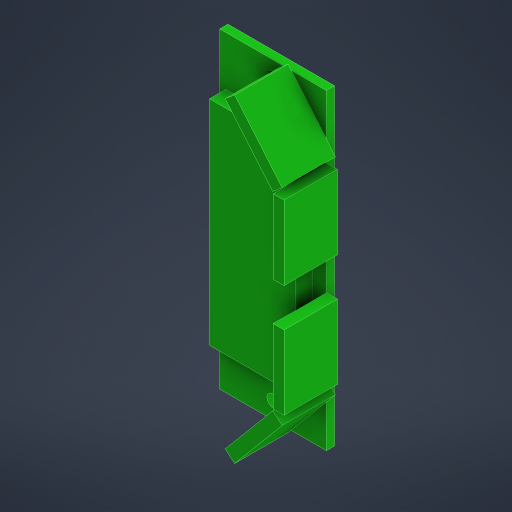
# Autodesk Inventor part: płytka_pcb
Saved by Autodesk Inventor 2023.4 (Build 274418000, 418)
## iProperties
Created: 2025-10-31
Part Number: płytka_pcb
Material: Tworzywo sztuczne ABS
Document SubType Name: Modeling
Designer: Jakub Borsukiewicz
Density: 1.06 g/cm^3
Appearance: Ciemnozielona
Author: Jakub Borsukiewicz
Autodesk Inventor part; units mm, degrees
ref_plane "YZ Plane" through (0, 0, 0) normal (1, 0, 0) x (0, 1, 0)
ref_plane "XZ Plane" through (0, 0, 0) normal (0, 1, 0) x (-1, 0, 0)
ref_plane "XY Plane" through (0, 0, 0) normal (0, 0, 1) x (1, 0, 0)
sketch "Szkic1" plane through (0, 0, 0) normal (0, 0, 1) x (1, 0, 0)
  line L0 (0, -7.6) -> (0, 45.6) projected
  line L1 (-5.2, 0) -> (31.2, 0) projected
  line L2 (0, 0) -> (26, 0)
  line L3 (26, 0) -> (26, 38)
  line L4 (26, 38) -> (0, 38)
  line L5 (0, 38) -> (0, 0)
  circle A0 centre (13, 34) radius 1.5
  point P0 (0, 38)
  dimension "d0" = 26
  dimension "d1" = 38
  dimension "d2" = 3
  dimension "d3" = 4
  dimension "d4" = 13
  constraints: 8 end point, 2 parallel, 1 centre point, 1 horizontal, 1 perpendicular
  measures "d0" distance of L3.end L4.end
  measures "d1" distance of L2.end L3.end
  measures "d2" diameter of A0
  measures "d3" distance from line of L4 A0.centre
  measures "d4" distance from line of L5 A0.centre
extrude "Wyciągnięcie proste1" add sketch "Szkic1" along normal blind 2
sketch "Szkic2" plane through (0, 0, 2) normal (0, 0, 1) x (1, 0, 0)
  line L0 (0, 38) -> (0, 0) projected
  line L1 (0, 0) -> (26, 0) projected
  line L2 (26, 0) -> (26, 38) projected
  line L3 (26, 38) -> (0, 38) projected
  circle A0 centre (13, 34) radius 1.5 projected
  line L4 (0, 0) -> (26, 0) projected
  line L5 (1.5, 0) -> (22.5, 0)
  line L6 (22.5, 0) -> (22.5, 26)
  line L7 (22.5, 26) -> (1.5, 26)
  line L8 (1.5, 26) -> (1.5, 0)
  dimension "d7" = 26
  dimension "d8" = 21
  dimension "d9" = 1.5
  constraints: 8 end point, 2 parallel, 1 horizontal, 1 perpendicular, 1 point on line
  measures "d7" distance of L5.end L6.end
  measures "d8" distance of L6.end L7.end
  measures "d9" distance between parallel lines of L0 L8
extrude "Wyciągnięcie proste2" add sketch "Szkic2" along normal blind 4 contours L8 L7 L6 L1
sketch "Szkic3" plane through (0, 0, 2) normal (0, 0, 1) x (1, 0, 0)
  line L0 (14.3427, 36.9572) -> (16.6412, 38.885)
  line L1 (16.6412, 38.885) -> (28.2083, 25.0936)
  line L2 (28.2083, 25.0936) -> (25.9097, 23.1658)
  line L3 (25.9097, 23.1658) -> (14.3427, 36.9572)
  line L4 (25.694, 22.676) -> (28.694, 22.676)
  line L5 (28.694, 22.676) -> (28.694, 4.676)
  line L6 (28.694, 4.676) -> (25.694, 4.676)
  line L7 (25.694, 4.676) -> (25.694, 22.676)
  line L8 (26, 0) -> (26, 38) projected
  point P0 (0, 0)
  point P1 (26, 22.676)
  point P2 (26, 4.676)
  dimension "d12" = 18
  dimension "d13" = 3
  dimension "d14" = 18
  dimension "d15" = 3
  constraints: 16 end point, 4 parallel, 3 perpendicular
  measures "d12" distance of L0.end L1.end
  measures "d13" distance of L1.end L2.end
  measures "d14" distance of L4.end L5.end
  measures "d15" distance of L5.end L6.end
extrude "Wyciągnięcie proste3" add sketch "Szkic3" along normal blind 13 contours L0 L1 L8 L2 L3 | L1 L2 L8 | L4 L5 L6 L8
mirror "Odbij1" about plane through (0, 0, 0) normal (0, 1, 0) of "Wyciągnięcie proste1", "Wyciągnięcie proste3", "Wyciągnięcie proste2"
